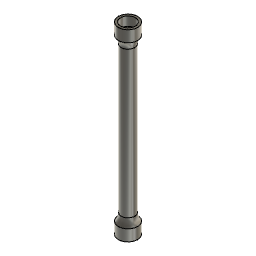
stuffing-tube (Autodesk Fusion 360 design; units mm, degrees)
Autodesk Fusion 360 part; units mm, degrees
sketch "Sketch1" plane through (0, 0, 0) normal (0, 0, 1) x (1, 0, 0)
  circle A0 centre (0, 0) radius 3
  dimension "d1" = 6
  constraint coincident A0.centre origin
  measures "d1" diameter of A0
extrude "Extrude1" add sketch "Sketch1" along normal blind 73
sketch "Sketch2" plane through (0, 0, 73) normal (0, 0, 1) x (-1, 0, 0)
  circle A0 centre (0, 0) radius 3
  circle A1 centre (0, 0) radius 2
  dimension "d4" = 4
  constraint concentric A0 A1
  measures "d4" diameter of A1
extrude "Extrude2" cut sketch "Sketch2" against normal blind 73 contours A1
sketch "Sketch3" plane through (0, 0, 73) normal (0, 0, 1) x (-1, 0, 0)
  circle A0 centre (0, 0) radius 2
  circle A1 centre (0, 0) radius 3
  circle A2 centre (0, 0) radius 4.25
  dimension "d7" = 8.5
  constraint concentric A0 A2
  measures "d7" diameter of A2
extrude "Extrude3" add sketch "Sketch3" along normal blind 4 and the other way blind 1 contours A1 | A2
sketch "Sketch4" plane through (0, 0, 77) normal (0, 0, 1) x (-1, 0, 0)
  circle A0 centre (0, 0) radius 2
  circle A1 centre (0, 0) radius 4.25
  circle A2 centre (0, 0) radius 3.25
  dimension "d10" = 6.5
  constraint coincident A0.centre A1.centre
  measures "d10" diameter of A2
extrude "Extrude4" cut sketch "Sketch4" against normal blind 4 contours A2
fillet "Fillet1" radius 5 1 edges at (-2.797, 1.0848, 72)
sketch "Sketch5" plane through (0, 0, 0) normal (0, 0, -1) x (1, 0, 0)
  circle A0 centre (0, 0) radius 2
  circle A1 centre (0, 0) radius 3
  circle A2 centre (0, 0) radius 4.25
  dimension "d16" = 8.5
  constraint concentric A0 A2
  measures "d16" diameter of A2
extrude "Extrude6" add sketch "Sketch5" along normal blind 4 and the other way blind 1 contours A1 | A2
sketch "Sketch6" plane through (0, 0, -4) normal (0, 0, -1) x (1, 0, 0)
  circle A0 centre (0, 0) radius 2
  circle A1 centre (0, 0) radius 4.25
  circle A2 centre (0, 0) radius 3.25
  dimension "d25" = 6.5
  constraint coincident A0.centre A1.centre
  measures "d25" diameter of A2
extrude "Extrude7" cut sketch "Sketch6" against normal blind 4 contours A2
fillet "Fillet2" radius 5 1 edges at (-2.797, -1.0848, 1)
